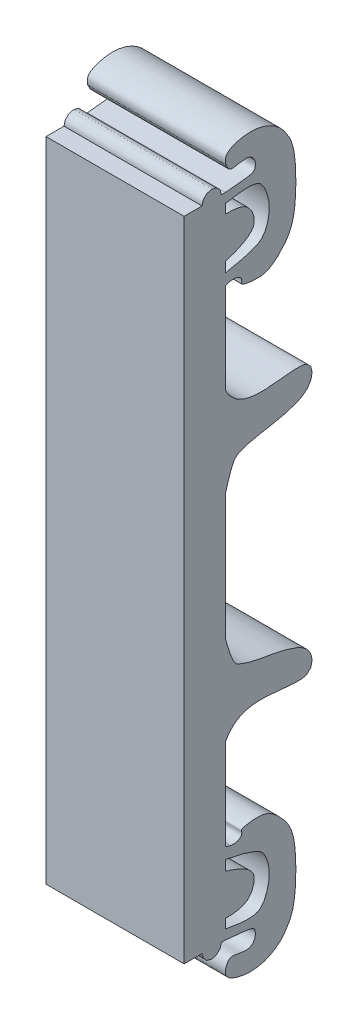
# Autodesk Inventor part: DIN-rail-mount
Saved by Autodesk Inventor 2023 (Build 270158030, 158C)
## iProperties
Created: 2024-03-20
Part Number: DIN-rail-mount
Material: Generic
Document SubType Name: Modeling
Designer: Imogen Heard
Density: 1 g/cm^3
Appearance: Default
Author: Imogen Heard
Autodesk Inventor part; units mm, degrees
ref_plane "YZ Plane" through (0, 0, 0) normal (1, 0, 0) x (0, 1, 0)
ref_plane "XZ Plane" through (0, 0, 0) normal (0, 1, 0) x (-1, 0, 0)
ref_plane "XY Plane" through (0, 0, 0) normal (0, 0, 1) x (1, 0, 0)
sketch "DIN-rail-clip-generic-V1.0" plane through (0, 0, 0) normal (0, 0, 1) x (1, 0, 0)
  line L0 (0, 40.9467) -> (3, 40.9467)
  line L1 (3, 40.9467) -> (3, 17.5)
  line L2 (3, 17.5) -> (0, 17.5)
  line L3 (0, 17.5) -> (0, 40.9467)
  line L4 (0, 35.1) -> (-0.3528, 35.269) construction
  line L5 (-0.3528, 35.269) -> (-1.1784, 35.269) construction
  line L6 (-1.1784, 35.269) -> (-1.277, 34.6657) construction
  line L7 (-1.277, 34.6657) -> (-0.9372, 34.5565) construction
  line L8 (-0.9372, 34.5565) -> (-2.5363, 34.2808) construction
  line L9 (-2.5363, 34.2808) -> (-3.3649, 34.5884) construction
  line L10 (-3.3649, 34.5884) -> (-4.7205, 35.8697) construction
  line L11 (-4.7205, 35.8697) -> (-5.1321, 37.4532) construction
  line L12 (-5.1321, 37.4532) -> (-5.1209, 40.8876) construction
  line L13 (-5.1209, 40.8876) -> (-4.7, 42.1113) construction
  line L14 (-4.7, 42.1113) -> (-3.9, 43.3113) construction
  line L15 (-3.9, 43.3113) -> (-2.1, 44.1113) construction
  line L16 (-2.1, 44.1113) -> (0, 43.5467) construction
  line L17 (0, 43.5467) -> (0.1036, 42.9467) construction
  line L18 (0.1036, 42.9467) -> (-0.2, 41.9467) construction
  line L19 (-0.2, 41.9467) -> (-1.1, 42.4004) construction
  line L20 (-1.1, 42.4004) -> (-2.3, 42.4379) construction
  spline S0 degree 4 poles (0, 35.1) (-0.3528, 35.269) (-1.1784, 35.269) (-1.277, 34.6657) (-0.9372, 34.5565) (-2.5363, 34.2808) (-3.3649, 34.5884) (-4.7205, 35.8697) (-5.1321, 37.4532) (-5.1209, 40.8876) (-4.7, 42.1113) (-3.9, 43.3113) (-2.1, 44.1113) (0, 43.5467) (0.1036, 42.9467) (-0.2, 41.9467) (-1.1, 42.4004) (-2.3, 42.4379) (-2.2829, 41.0379) (-1.7552, 41.1368) (0, 40.9467) knots 1 1 1 1 1 2 3 4 5 6 7 8 9 10 11 12 13 14 15 16 17 17.993985 17.993985 17.993985 17.993985 17.993985
  line L21 (0, 35.8905) -> (-0.7907, 36.0877) construction
  line L22 (-0.7907, 36.0877) -> (-1.1784, 36.0877) construction
  line L23 (-1.1784, 36.0877) -> (-2.2779, 36.5342) construction
  line L24 (-2.2779, 36.5342) -> (-2.7458, 36.6343) construction
  line L25 (-2.7458, 36.6343) -> (-3.471, 38.3527) construction
  line L26 (-3.471, 38.3527) -> (-2.7458, 40.1075) construction
  spline S1 degree 4 poles (0, 35.8905) (-0.7907, 36.0877) (-1.1784, 36.0877) (-2.2779, 36.5342) (-2.7458, 36.6343) (-3.471, 38.3527) (-2.7458, 40.1075) (-2.4429, 40.6075) (-0.7055, 40.4056) (0, 40.2568) knots 1 1 1 1 1 2 3 4 5 6 6.977977 6.977977 6.977977 6.977977 6.977977
  line L27 (-2.3, 42.4379) -> (-2.2829, 41.0379) construction
  line L28 (-2.2829, 41.0379) -> (-1.7552, 41.1368) construction
  line L29 (-1.7552, 41.1368) -> (0, 40.9467) construction
  line L30 (-2.7458, 40.1075) -> (-2.4429, 40.6075) construction
  line L31 (-2.4429, 40.6075) -> (-0.7055, 40.4056) construction
  line L32 (-0.7055, 40.4056) -> (0, 40.2568) construction
  line L33 (0, 36.6343) -> (-1.1784, 36.9758) construction
  line L34 (-1.1784, 36.9758) -> (-2.2101, 37.6402) construction
  line L35 (-2.2101, 37.6402) -> (-2.1452, 38.3006) construction
  line L36 (-2.1452, 38.3006) -> (-1.8076, 39.3817) construction
  line L37 (-1.8076, 39.3817) -> (-0.8778, 39.5886) construction
  line L38 (-0.8778, 39.5886) -> (0, 39.5886) construction
  spline S2 degree 4 poles (0, 36.6343) (-1.1784, 36.9758) (-2.2101, 37.6402) (-2.1452, 38.3006) (-1.8076, 39.3817) (-0.8778, 39.5886) (0, 39.5886) knots 1 1 1 1 1 2 3 4 4 4 4 4
  line L39 (-0.5144, 23.8721) -> (0, 22.0778) construction
  spline S3 degree 4 poles (0, 28.5164) (-0.0002, 28.5161) (-0.1764, 28.1682) (-0.5144, 27.8581) (-1.1668, 26.9412) (-3.3762, 27.1074) (-5.9868, 27.5396) (-6.4206, 26.5054) (-5.8606, 24.9054) (-2.8606, 24.6412) (-1.4606, 24.4656) (-0.5144, 23.8721) (0, 22.0778) knots 1 1 1 1 1 1.050464 1.110527 1.512977 1.739488 1.83789 2 2.236311 2.876473 3 3 3 3 3
  line L40 (-1.4606, 24.4656) -> (-0.5144, 23.8721) construction
  line L41 (-3.3762, 27.1074) -> (-5.9868, 27.5396) construction
  line L42 (-5.9868, 27.5396) -> (-6.4206, 26.5054) construction
  line L43 (-6.4206, 26.5054) -> (-5.8606, 24.9054) construction
  line L44 (-5.8606, 24.9054) -> (-2.8606, 24.6412) construction
  line L45 (-2.8606, 24.6412) -> (-1.4606, 24.4656) construction
  line L46 (0, 28.5164) -> (-0.1764, 28.1682) construction
  line L47 (-0.1764, 28.1682) -> (-0.5144, 27.8581) construction
  line L48 (-0.5144, 27.8581) -> (-1.1668, 26.9412) construction
  line L49 (-1.1668, 26.9412) -> (-3.3762, 27.1074) construction
  circle A0 centre (1, 40.9467) radius 0.7
  point P0 (0, 17.5)
  point P1 (-0.5, 35)
  point P2 (-1, 33.6)
  dimension "d63" = 3
  dimension "d68" = 23.4467
  dimension "d71" = 0.9373
  dimension "d73" = 0.269
  dimension "d74" = 0.3528
  dimension "d79" = 1.5363
  dimension "d85" = 0.7905
  dimension "d87" = 1.1784
  dimension "d88" = 0.7907
  dimension "d89" = 1.5835
  dimension "d90" = 5.1321
  dimension "d92" = 2.2779
  dimension "d93" = 2.7458
  dimension "d95" = 1.7184
  dimension "d96" = 0.7252
  dimension "d97" = 3.4344
  dimension "d99" = 1.2236
  dimension "d100" = 0.4209
  dimension "d101" = 1.2
  dimension "d102" = 0.8
  dimension "d103" = 1.8
  dimension "d104" = 0.8
  dimension "d105" = 2.6
  dimension "d106" = 0.1036
  dimension "d107" = 2
  dimension "d108" = 0.2
  dimension "d109" = 1
  dimension "d110" = 0.9
  dimension "d111" = 0.4536
  dimension "d112" = 1.2
  dimension "d113" = 1.4
  dimension "d114" = 0.0375
  dimension "d115" = 0.0171
  dimension "d116" = 0.5278
  dimension "d117" = 0.0989
  dimension "d118" = 0.69
  dimension "d119" = 0.6682
  dimension "d120" = 0.7055
  dimension "d121" = 0.5412
  dimension "d122" = 1.7374
  dimension "d123" = 0.2019
  dimension "d124" = 0.5
  dimension "d125" = 0.3029
  dimension "d126" = 1.1784
  dimension "d127" = 3.9709
  dimension "d128" = 0.6643
  dimension "d129" = 1.0316
  dimension "d130" = 0.6604
  dimension "d131" = 0.0649
  dimension "d132" = 1.8076
  dimension "d133" = 1.565
  dimension "d134" = 0.9298
  dimension "d136" = 0.7438
  dimension "d138" = 0.3482
  dimension "d139" = 0.3101
  dimension "d140" = 0.9169
  dimension "d141" = 2.2093
  dimension "d142" = 0.1662
  dimension "d143" = 0.1764
  dimension "d144" = 0.3381
  dimension "d145" = 0.6524
  dimension "d147" = 0.4338
  dimension "d148" = 1.6
  dimension "d149" = 0.56
  measures "d63" distance of the line from the sketch origin of L1
  measures "d68" distance between parallel lines of L2 L0
  measures "d73" vertical distance of L4.end point (-0.5, 35)
  measures "d79" horizontal distance of point (-1, 33.6) L8.end
  measures "d85" distance of L21.start L4.start
  measures "d89" vertical distance of L10.end L11.end
  measures "d95" vertical distance of L24.end L25.end
  measures "d96" horizontal distance of L25.end L24.end
  measures "d97" distance of L11.end L12.end
  measures "d99" vertical distance of L12.end L13.end
  measures "d100" horizontal distance of L13.end L12.end
  measures "d101" vertical distance of L14.end L13.end
  measures "d102" horizontal distance of L14.end L13.end
  measures "d103" horizontal distance of L15.end L14.end
  measures "d104" vertical distance of L14.end L15.end
  measures "d105" distance from line of L0 L16.end
  measures "d107" distance from line of L0 L17.end
  measures "d109" distance from line of L0 L18.end
  measures "d110" horizontal distance of L18.end L19.end
  measures "d111" vertical distance of L18.end L19.end
  measures "d112" horizontal distance of L19.end L20.end
  measures "d113" vertical distance of L27.end L20.end
  measures "d114" vertical distance of L20.end L19.end
  measures "d115" horizontal distance of L20.end L27.end
  measures "d116" horizontal distance of L27.end L28.end
  measures "d117" vertical distance of L27.end L28.end
  measures "d118" distance of L29.end L32.end
  measures "d119" distance of L38.end L32.end
  measures "d121" distance from line of L31.end L0
  measures "d122" horizontal distance of L30.end L31.end
  measures "d123" vertical distance of L30.end L31.end
  measures "d124" vertical distance of L26.end L30.end
  measures "d125" horizontal distance of L30.end L26.end
  measures "d127" distance from line of L0 L33.end
  measures "d128" vertical distance of L33.end L34.end
  measures "d129" horizontal distance of L33.end L34.end
  measures "d130" vertical distance of L35.end L34.end
  measures "d131" horizontal distance of L35.end L34.end
  measures "d133" distance from line of L36.end L0
  measures "d134" horizontal distance of L36.end L37.end
  measures "d136" distance of L21.start L33.start
  measures "d138" vertical distance of point (0, 28.516) L46.end
  measures "d139" vertical distance of L46.end L47.end
  measures "d140" vertical distance of L47.end L48.end
  measures "d141" horizontal distance of L49.end L48.end
  measures "d142" vertical distance of L48.end L49.end
  measures "d143" horizontal distance of L46.end point (0, 28.516)
  measures "d144" horizontal distance of L47.end L46.end
  measures "d145" horizontal distance of L47.end L48.end
  measures "d147" horizontal distance of L42.end L41.end
  measures "d148" vertical distance of L42.end L43.end
  measures "d149" horizontal distance of L43.end L42.end
sketch "Sketch1" plane through (0, 0, 0) normal (1, 0, 0) x (0, 1, 0)
  line L0 (5.8, -7.3) -> (29.2, -7.3)
  line L1 (29.2, -6.3) -> (5.8, -6.3)
  line L2 (32.2, -1) -> (35, -1)
  line L3 (35, -1) -> (35, 0)
  line L4 (35, 0) -> (32.2, 0)
  line L5 (-1817770.1114, -20.3632) -> (-1817770.1114, -1)
  line L6 (2.8, 0) -> (0, 0)
  line L7 (0, 0) -> (0, -1)
  line L8 (0, -1) -> (2.8, -1)
  line L9 (4.8, -2) -> (4.8, -5.3)
  arc A0 (32.2, -1) -> (31.2, -2) centre (32.2, -2) ccw
  arc A1 (29.2, -6.3) -> (30.2, -5.3) centre (29.2, -5.3) ccw
  arc A2 (4.8, -5.3) -> (5.8, -6.3) centre (5.8, -5.3) ccw
  arc A3 (3.8, -2) -> (2.8, -1) centre (2.8, -2) ccw
  arc A4 (4.8, -2) -> (2.8, 0) centre (2.8, -2) ccw
  arc A5 (3.8, -5.3) -> (5.8, -7.3) centre (5.8, -5.3) ccw
  line L10 (3.8, -2) -> (3.8, -5.3)
  arc A6 (32.2, 0) -> (30.2, -2) centre (32.2, -2) ccw
  arc A7 (29.2, -7.3) -> (31.2, -5.3) centre (29.2, -5.3) ccw
  line L11 (31.2, -2) -> (31.2, -5.3)
  line L12 (30.2, -2) -> (30.2, -5.3)
  line L13 (17.5, -4.8951) -> (17.5, -40.6352) construction
  point P0 (4.8, -3.65)
  dimension "d0" = 1
  dimension "d1" = 1
  dimension "d5" = 35
  dimension "d8" = 7.3
  dimension "d9" = 1
  dimension "d10" = 1
  dimension "d11" = 2
  dimension "d12" = 2
  dimension "d13" = 12.7
  dimension "d15" = 12.7
  dimension "d16" = 4.8
  dimension "d17" = 4.8
  dimension "d20" = 1
  dimension "d21" = 1
  dimension "d22" = 2
  constraints: 28 end point, 17 point on circle, 12 tangent, 8 centre point, 7 horizontal alignment, 4 equal radius, 4 parallel, 3 perpendicular, 2 horizontal, 2 vertical, 1 coincident, 1 midpoint, 1 point on line, 1 vertical alignment
  measures "d0" distance between parallel lines of L2 L4
  measures "d1" distance between parallel lines of L0 L1
  measures "d5" distance between parallel lines of L7 L3
  measures "d8" distance between parallel lines of L4 L0
  measures "d9" radius of A0
  measures "d10" radius of A1
  measures "d11" radius of A4
  measures "d12" radius of A6
  measures "d13" distance between parallel lines of L13 L12
  measures "d15" distance between parallel lines of L13 L9
  measures "d16" distance between parallel lines of L9 L7
  measures "d17" distance between parallel lines of L12 L3
  measures "d20" distance between parallel lines of L12 L11
  measures "d21" distance between parallel lines of L10 L9
  measures "d22" radius of A5
sketch "Sketch4" plane through (0, 0, 0) normal (-1, 0, 0) x (0, 0, 1)
  line L0 (-1, 32.2) -> (-1, 35) projected
  line L1 (-1, 35) -> (0, 35) projected
  line L2 (0, 35) -> (0, 32.2) projected
  line L3 (-4.8951, 17.5) -> (-40.6352, 17.5) construction
  line L4 (-2, 31.2) -> (-5.3, 31.2) projected
  line L5 (-2, 30.2) -> (-5.3, 30.2) projected
  line L6 (-7.3, 5.8) -> (-7.3, 29.2) projected
  line L7 (-6.3, 29.2) -> (-6.3, 5.8) projected
  line L8 (-2, 3.8) -> (-5.3, 3.8) projected
  line L9 (-2, 4.8) -> (-5.3, 4.8) projected
  line L10 (-1, 0) -> (-1, 2.8) projected
  line L11 (0, 2.8) -> (0, 0) projected
  line L12 (0, 0) -> (-1, 0) projected
  line L13 (0, 40.9467) -> (3, 40.9467)
  line L14 (3, 40.9467) -> (3, 17.5)
  line L15 (3, 17.5) -> (0, 17.5)
  line L16 (0, 17.5) -> (0, 40.9467)
  line L17 (0, 35.1) -> (-0.3528, 35.269) construction
  line L18 (-0.3528, 35.269) -> (-1.1784, 35.269) construction
  line L19 (-1.1784, 35.269) -> (-1.277, 34.6657) construction
  line L20 (-1.277, 34.6657) -> (-0.9372, 34.5565) construction
  line L21 (-0.9372, 34.5565) -> (-2.5363, 34.2808) construction
  line L22 (-2.5363, 34.2808) -> (-3.3649, 34.5884) construction
  line L23 (-3.3649, 34.5884) -> (-4.7205, 35.8697) construction
  line L24 (-4.7205, 35.8697) -> (-5.1321, 37.4532) construction
  line L25 (-5.1321, 37.4532) -> (-5.1209, 40.8876) construction
  line L26 (-5.1209, 40.8876) -> (-4.7, 42.1113) construction
  line L27 (-4.7, 42.1113) -> (-3.9, 43.3113) construction
  line L28 (-3.9, 43.3113) -> (-2.1, 44.1113) construction
  line L29 (-2.1, 44.1113) -> (0, 43.5467) construction
  line L30 (0, 43.5467) -> (0.1036, 42.9467) construction
  line L31 (0.1036, 42.9467) -> (-0.2, 41.9467) construction
  line L32 (-0.2, 41.9467) -> (-1.1, 42.4004) construction
  line L33 (-1.1, 42.4004) -> (-2.3, 42.4379) construction
  spline S0 degree 4 poles (0, 35.1) (-0.3528, 35.269) (-1.1784, 35.269) (-1.277, 34.6657) (-0.9372, 34.5565) (-2.5363, 34.2808) (-3.3649, 34.5884) (-4.7205, 35.8697) (-5.1321, 37.4532) (-5.1209, 40.8876) (-4.7, 42.1113) (-3.9, 43.3113) (-2.1, 44.1113) (0, 43.5467) (0.1036, 42.9467) (-0.2, 41.9467) (-1.1, 42.4004) (-2.3, 42.4379) (-2.2829, 41.0379) (-1.7552, 41.1368) (0, 40.9467) knots 1 1 1 1 1 2 3 4 5 6 7 8 9 10 11 12 13 14 15 16 17 17.993985 17.993985 17.993985 17.993985 17.993985
  line L34 (0, 35.8905) -> (-0.7907, 36.0877) construction
  line L35 (-0.7907, 36.0877) -> (-1.1784, 36.0877) construction
  line L36 (-1.1784, 36.0877) -> (-2.2779, 36.5342) construction
  line L37 (-2.2779, 36.5342) -> (-2.7458, 36.6343) construction
  line L38 (-2.7458, 36.6343) -> (-3.471, 38.3527) construction
  line L39 (-3.471, 38.3527) -> (-2.7458, 40.1075) construction
  spline S1 degree 4 poles (0, 35.8905) (-0.7907, 36.0877) (-1.1784, 36.0877) (-2.2779, 36.5342) (-2.7458, 36.6343) (-3.471, 38.3527) (-2.7458, 40.1075) (-2.4429, 40.6075) (-0.7055, 40.4056) (0, 40.2568) knots 1 1 1 1 1 2 3 4 5 6 6.977977 6.977977 6.977977 6.977977 6.977977
  line L40 (-2.3, 42.4379) -> (-2.2829, 41.0379) construction
  line L41 (-2.2829, 41.0379) -> (-1.7552, 41.1368) construction
  line L42 (-1.7552, 41.1368) -> (0, 40.9467) construction
  line L43 (-2.7458, 40.1075) -> (-2.4429, 40.6075) construction
  line L44 (-2.4429, 40.6075) -> (-0.7055, 40.4056) construction
  line L45 (-0.7055, 40.4056) -> (0, 40.2568) construction
  line L46 (0, 36.6343) -> (-1.1784, 36.9758) construction
  line L47 (-1.1784, 36.9758) -> (-2.2101, 37.6402) construction
  line L48 (-2.2101, 37.6402) -> (-2.1452, 38.3006) construction
  line L49 (-2.1452, 38.3006) -> (-1.8076, 39.3817) construction
  line L50 (-1.8076, 39.3817) -> (-0.8778, 39.5886) construction
  line L51 (-0.8778, 39.5886) -> (0, 39.5886) construction
  spline S2 degree 4 poles (0, 36.6343) (-1.1784, 36.9758) (-2.2101, 37.6402) (-2.1452, 38.3006) (-1.8076, 39.3817) (-0.8778, 39.5886) (0, 39.5886) knots 1 1 1 1 1 2 3 4 4 4 4 4
  line L52 (-0.5144, 23.8721) -> (0, 22.0778) construction
  spline S3 degree 4 poles (0, 28.5164) (-0.0002, 28.5161) (-0.1764, 28.1682) (-0.5144, 27.8581) (-1.1668, 26.9412) (-3.3762, 27.1074) (-5.9868, 27.5396) (-6.4206, 26.5054) (-5.8606, 24.9054) (-2.8606, 24.6412) (-1.4606, 24.4656) (-0.5144, 23.8721) (0, 22.0778) knots 1 1 1 1 1 1.050464 1.110527 1.512977 1.739488 1.83789 2 2.236311 2.876473 3 3 3 3 3
  line L53 (-1.4606, 24.4656) -> (-0.5144, 23.8721) construction
  line L54 (-3.3762, 27.1074) -> (-5.9868, 27.5396) construction
  line L55 (-5.9868, 27.5396) -> (-6.4206, 26.5054) construction
  line L56 (-6.4206, 26.5054) -> (-5.8606, 24.9054) construction
  line L57 (-5.8606, 24.9054) -> (-2.8606, 24.6412) construction
  line L58 (-2.8606, 24.6412) -> (-1.4606, 24.4656) construction
  line L59 (0, 28.5164) -> (-0.1764, 28.1682) construction
  line L60 (-0.1764, 28.1682) -> (-0.5144, 27.8581) construction
  line L61 (-0.5144, 27.8581) -> (-1.1668, 26.9412) construction
  line L62 (-1.1668, 26.9412) -> (-3.3762, 27.1074) construction
  circle A0 centre (1, 40.9467) radius 0.7
  point P0 (1.7, 40.9467)
  point P1 (0.3, 40.9467)
  constraints: 1 horizontal, 1 vertical, 1 other
extrude "Extrusion4" add sketch "Sketch4" against normal blind 10 contours L16 L13 A0 L14 L15 L2 | S0 L16 S1 | L16 S3 | S2 L16 | A0 L13 | L13 A0
mirror "Mirror1" about plane through (0, 17.5, 3) normal (0, -1, 0)
ref_plane "Work Plane1" through (10, 7.3119, 10.62) normal (1, 0, 0) x (0, -1, 0)
sketch "din-rail-clip-outline" plane through (10, 7.3119, 10.62) normal (1, 0, 0) x (0, -1, 0)
  line L0 (11.9005, 10.62) -> (12.5687, 10.62) projected
  line L1 (8.2025, 10.62) -> (8.9463, 10.62) projected
  line L2 (-14.7658, 10.62) -> (-5.6103, 10.62) projected
  line L3 (-21.2045, 10.62) -> (-27.7881, 10.62) projected
  line L4 (-33.6348, 10.62) -> (-33.6348, 10.32) projected
  line L5 (-33.6348, 7.62) -> (13.2587, 7.62) projected
  line L6 (13.2587, 10.62) -> (13.2587, 10.32) projected
  line L7 (0.8284, 10.62) -> (7.4119, 10.62) projected
  line L8 (-28.5786, 10.62) -> (-29.3224, 10.62) projected
  line L9 (-32.2766, 10.62) -> (-32.9448, 10.62) projected
  arc A0 (-33.6348, 10.32) -> (-33.6348, 8.92) centre (-33.6348, 9.62) ccw projected
  line L10 (-33.6348, 8.92) -> (-33.6348, 7.62) projected
  line L11 (13.2587, 8.92) -> (13.2587, 7.62) projected
  arc A1 (13.2587, 8.92) -> (13.2587, 10.32) centre (13.2587, 9.62) ccw projected
  point P0 (7.3119, 10.62)
  constraints: 8 horizontal alignment
sketch "Sketch3" plane through (0, 41.284, -13.8819) normal (0, 0, 1) x (1, 0, 0)
  line L0 (110, 34.2) -> (302, 34.2)
  line L1 (302, 34.2) -> (302, -10.8)
  line L2 (302, -10.8) -> (110, -10.8)
  line L3 (110, -10.8) -> (110, 34.2)
  line L4 (0, 23.4) -> (0, 0) projected
  line L5 (300, 23.4) -> (300, 0) projected
  line L6 (0, -5.8) -> (300, -5.8) projected
  line L7 (0, 29.2) -> (300, 29.2) projected
  point P0 (0, -41.284)
  dimension "d56" = 110
  dimension "d57" = 2
  dimension "d58" = 5
  dimension "d59" = 5
  constraints: 8 end point, 2 parallel, 1 horizontal, 1 perpendicular
  measures "d56" distance between parallel lines of L4 L3
  measures "d57" distance between parallel lines of L5 L1
  measures "d58" distance between parallel lines of L2 L6
  measures "d59" distance between parallel lines of L0 L7
